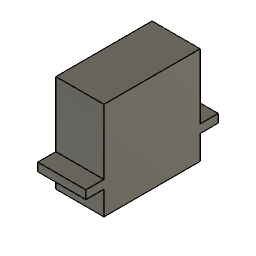
サーボモータ模型 (Autodesk Fusion 360 design; units mm, degrees)
Autodesk Fusion 360 part; units mm, degrees
sketch "スケッチ1" plane through (0, 0, 0) normal (0, 0, 1) x (1, 0, 0)
  line L0 (0, 0) -> (20, 0)
  line L1 (20, 0) -> (20, 40)
  line L2 (20, 40) -> (0, 40)
  line L3 (0, 40) -> (0, 0)
  dimension "d1" = 20
  dimension "d2" = 40
  constraint horizontal L0
  constraint vertical L1
  constraint horizontal L2
  constraint vertical L3
  constraint coincident L0.start L3.end
  measures "d1" distance of L1.end L2.end
  measures "d2" distance of L0.start L2.end
extrude "押し出し1" add sketch "スケッチ1" along normal blind 10
sketch "スケッチ2" plane through (0, 0, 10) normal (0, 0, 1) x (-1, 0, 0)
  line L0 (0, -40) -> (0, 0)
  line L1 (0, 0) -> (-20, 0)
  line L2 (-20, 0) -> (-20, -40)
  line L3 (-20, -40) -> (0, -40)
  line L4 (0, -47.5) -> (-20, -47.5)
  line L5 (-20, -47.5) -> (-20, 7.5)
  line L6 (-20, 7.5) -> (0, 7.5)
  line L7 (0, 7.5) -> (0, -47.5)
  dimension "d5" = 55
  dimension "d6" = 7.5
  constraint horizontal L4
  constraint vertical L5
  constraint horizontal L6
  constraint vertical L7
  measures "d5" distance of L4.start L6.end
  measures "d6" distance of L3 L4
extrude "押し出し2" add sketch "スケッチ2" along normal blind 3.5
sketch "スケッチ3" plane through (0, 0, 13.5) normal (0, 0, 1) x (-1, 0, 0)
  line L0 (0, 7.5) -> (-20, 7.5)
  line L1 (-20, 7.5) -> (-20, -47.5)
  line L2 (-20, -47.5) -> (0, -47.5)
  line L3 (0, -47.5) -> (0, 7.5)
  line L4 (0, 0) -> (-20, 0)
  line L5 (-20, 0) -> (-20, -40)
  line L6 (-20, -40) -> (0, -40)
  line L7 (0, -40) -> (0, 0)
  dimension "d9" = 40
  constraint horizontal L4
  constraint vertical L5
  constraint horizontal L6
  constraint vertical L7
  constraint coincident L1 L5.end
  constraint coincident L4.start L7.end
  measures "d9" distance of L4.end L5.end
extrude "押し出し3" add sketch "スケッチ3" along normal blind 27 contours L1 L3 L4 L5 L6 L7
sketch "スケッチ4" plane through (0, 0, 0) normal (0, 0, -1) x (1, 0, 0)
  line L0 (0, 0) -> (0, -40)
  line L1 (0, -40) -> (20, -40)
  line L2 (20, -40) -> (20, 0)
  line L3 (20, 0) -> (0, 0)
  circle A0 centre (10, -10) radius 3
  dimension "d12" = 6
  measures "d12" diameter of A0
extrude "押し出し4" add sketch "スケッチ4" along normal blind 6.5 contours A0
